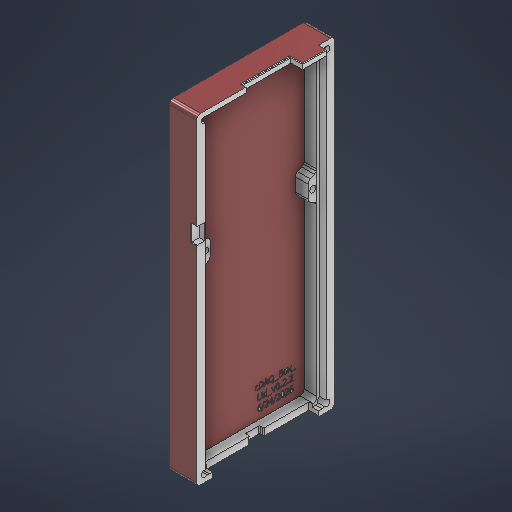
# Autodesk Inventor part: cDAQ_Box_Lid_v0.2.3
Saved by Autodesk Inventor 2027 (Build 310192000, 192)
## iProperties
Created: 2026-05-08
Part Number: cDAQ_Box_Lid_v0.2.3
Material: Generic
Document SubType Name: Modeling
Designer: giese
Density: 1 g/cm^3
Appearance: Default
Author: giese
Autodesk Inventor part; units mm, degrees
(part 1 of 2)
ref_plane "YZ Plane" through (0, 0, 0) normal (1, 0, 0) x (0, 1, 0)
ref_plane "XZ Plane" through (0, 0, 0) normal (0, 1, 0) x (-1, 0, 0)
ref_plane "XY Plane" through (0, 0, 0) normal (0, 0, 1) x (1, 0, 0)
sketch "Sketch1" plane through (0, 0, 0) normal (1, 0, 0) x (0, 1, 0)
  line L0 (50.7569, 48.4212) -> (-204.2591, 48.4212)
  line L1 (-204.2591, 48.4212) -> (-204.2591, -60.7988)
  line L2 (-204.2591, -60.7988) -> (50.7569, -60.7988)
  line L3 (50.7569, -60.7988) -> (50.7569, 48.4212)
  point P0 (0, 0)
  dimension "d0" = 109.22
  dimension "d1" = 255.016
  constraints: 8 end point, 2 parallel, 1 horizontal, 1 perpendicular
  measures "d0" distance of L2.end L0.start
  measures "d1" distance of L0.start L0.end
extrude "Extrusion1" add sketch "Sketch1" along normal blind 21.59
sketch "Sketch2" plane through (21.59, 0, 0) normal (1, 0, 0) x (0, 0, -1)
  line L0 (-39.5312, 44.4069) -> (51.9088, 44.4069)
  line L1 (51.9088, 44.4069) -> (51.9088, -197.9091)
  line L2 (51.9088, -197.9091) -> (-39.5312, -197.9091)
  line L3 (-39.5312, -197.9091) -> (-39.5312, 44.4069)
  line L4 (-48.4212, 50.7569) -> (-48.4212, -204.2591) projected
  line L5 (-48.4212, -204.2591) -> (60.7988, -204.2591) projected
  line L6 (60.7988, -204.2591) -> (60.7988, 50.7569) projected
  point P0 (0, 0)
  dimension "d4" = 91.44
  dimension "d5" = 242.316
  dimension "d6" = 8.89
  dimension "d7" = 6.35
  dimension "d226" = 8.89
  constraints: 8 end point, 2 parallel, 1 horizontal, 1 perpendicular
  measures "d4" distance of L0.start L0.end
  measures "d5" distance of L0.end L1.end
  measures "d6" distance between parallel lines of L4 L3
  measures "d7" distance between parallel lines of L5 L2
  measures "d226" distance between parallel lines of L6 L1
extrude "Extrusion2" cut sketch "Sketch2" against normal blind 15.24
sketch "Sketch3" plane through (0, 0, 0) normal (-1, 0, 0) x (0, 0, 1)
  circle A0 centre (-37.9388, 7.3229) radius 2
  line L0 (-60.7988, -204.2591) -> (-60.7988, 50.7569) projected
  line L1 (-60.7988, 50.7569) -> (48.4212, 50.7569) projected
  circle A1 centre (-19.44, 7.3229) radius 2
  circle A2 centre (-0.9411, 7.3229) radius 2
  point P0 (0, 0)
  dimension "d10" = 22.86
  dimension "d11" = 43.434
  dimension "d12" = 43.434
  dimension "d13" = 18.4988
  dimension "d14" = 4
  dimension "d15" = 4
  dimension "d16" = 43.434
  dimension "d17" = 18.4988
  dimension "d18" = 36.9976
  dimension "d21" = 4
  constraints: 3 centre point
  measures "d10" distance from line of L0 A0.centre
  measures "d11" distance from line of L1 A0.centre
  measures "d12" distance from line of L1 A1.centre
  measures "d13" distance of A0.centre A1.centre
  measures "d14" diameter of A1
  measures "d15" diameter of A2
  measures "d16" distance from line of L1 A2.centre
  measures "d17" distance of A1.centre A2.centre
  measures "d18" distance of A0.centre A2.centre
  measures "d21" diameter of A0
extrude "Extrusion3" [suppressed]
sketch "Sketch6" plane through (0, 50.7569, 48.4212) normal (0, 1, 0) x (1, 0, 0)
  line L0 (21.59, 8.89) -> (21.59, 100.33) projected
  line L1 (17.78, 39.37) -> (21.59, 39.37)
  line L2 (21.59, 39.37) -> (21.59, 96.52)
  line L3 (21.59, 96.52) -> (17.78, 96.52)
  line L4 (17.78, 96.52) -> (17.78, 39.37)
  line L5 (0, 109.22) -> (21.59, 109.22) projected
  point P0 (0, 48.4212)
  point P1 (21.59, 39.37)
  point P2 (19.685, 96.52)
  point P3 (19.685, 39.37)
  dimension "d30" = 3.81
  dimension "d32" = 12.7
  dimension "d220" = 69.85
  constraints: 8 end point, 2 midpoint, 2 parallel, 1 horizontal, 1 perpendicular, 1 point on line
  measures "d30" distance between parallel lines of L0 L4
  measures "d32" distance between parallel lines of L5 L3
  measures "d220" distance between parallel lines of L5 L1
extrude "Extrusion5" cut sketch "Sketch6" against normal blind 6.35
fillet "Fillet1" radius 3.175 4 edges at (10.795, 50.7569, -60.7988) (10.795, 50.7569, 48.4212) (10.795, -204.2591, 48.4212) (10.795, -204.2591, -60.7988)
sketch "Sketch7" plane through (21.59, 0, 0) normal (1, 0, 0) x (0, 0, -1)
  line L0 (-39.5312, -197.9091) -> (-39.5312, 44.4069) projected
  line L1 (-39.5312, 44.4069) -> (-42.3252, 44.4069)
  line L2 (-42.3252, 46.6929) -> (-41.6902, 46.6929)
  line L3 (-41.6902, 46.6929) -> (-41.6902, 51.0109)
  line L4 (-39.5312, -190.1621) -> (-39.5312, -197.9091)
  line L5 (51.9088, -197.9091) -> (-39.5312, -197.9091) projected
  line L6 (-40.4202, -200.1951) -> (-41.6902, -200.1951)
  line L7 (-41.6902, -200.1951) -> (-41.6902, -190.1621)
  line L8 (51.9088, 44.4069) -> (51.9088, -197.9091) projected
  line L9 (51.9088, -192.7021) -> (51.9088, -197.9091)
  line L10 (51.9088, -197.9091) -> (43.9078, -197.9091)
  line L11 (51.9088, -197.9091) -> (51.9088, -192.7021)
  line L12 (54.0678, -192.7021) -> (54.0678, -200.1951)
  line L13 (54.0678, -200.1951) -> (43.9078, -200.1951)
  line L14 (-39.5312, 44.4069) -> (51.9088, 44.4069) projected
  line L15 (42.0028, 44.4069) -> (51.9088, 44.4069)
  line L16 (54.0678, 48.4709) -> (54.0678, 46.6929)
  line L17 (54.0678, 46.6929) -> (42.0028, 46.6929)
  line L18 (-42.3252, 46.6929) -> (42.0028, 46.6929)
  line L19 (42.0028, 44.4069) -> (-42.3252, 44.4069)
  line L20 (54.0678, 48.4709) -> (54.0678, -192.7021)
  line L21 (44.2888, -195.2421) -> (44.2888, 44.4069)
  line L22 (43.9078, -197.9091) -> (-40.4202, -197.9091)
  line L23 (-40.4202, -200.1951) -> (43.9078, -200.1951)
  line L24 (-41.6902, -190.1621) -> (-41.6902, 51.0109)
  line L25 (-39.5312, 44.4069) -> (-39.5312, -190.1621)
  point P0 (0, 0)
  point P1 (-39.5312, 51.0109)
  point P2 (-44.2302, 48.9789)
  point P3 (51.9088, 48.4709)
  point P4 (54.0678, 46.6929)
  point P5 (-42.0712, 50.7569)
  point P6 (49.3688, 50.7569)
  point P7 (-44.2302, -190.0351)
  point P8 (51.5278, -190.0351)
  point P9 (-41.6902, 46.6929)
  dimension "d34" = 2.286
  dimension "d35" = 2.159
  dimension "d38" = 2.159
  dimension "d39" = 2.286
  dimension "d42" = 2.286
  dimension "d43" = 2.159
  dimension "d46" = 2.286
  dimension "d47" = 2.159
  constraints: 44 end point, 5 point on line, 4 parallel, 4 perpendicular, 2 collinear, 2 horizontal, 2 vertical, 6 other
  measures "d34" distance between parallel lines of L2 L1
  measures "d39" distance between parallel lines of L5 L6
  measures "d42" distance between parallel lines of L5 L13
  measures "d46" distance between parallel lines of L14 L17
extrude "Extrusion6" cut sketch "Sketch7" against normal blind 5 contours L0 L14 L8 L5 | L6 L7 L24 L18 L17 L20 L12 L13 L23
fillet "Fillet2" radius 3.175 6 edges at (11.47, 44.4069, 39.5312) (11.47, 44.4069, -51.9088) (11.47, -197.9091, 39.5312) (19.09, -200.1951, 41.6902) (11.47, -197.9091, -51.9088) (19.09, -200.1951, -54.0678)
sketch "Sketch11" plane through (16.59, 0, 0) normal (1, 0, 0) x (0, 0, -1)
  circle A0 centre (54.7028, 44.6609) radius 2.4005
  line L0 (57.6238, 50.7569) -> (48.0988, 50.7569) projected
  line L1 (60.7988, -201.0841) -> (60.7988, 47.5819) projected
  arc A1 (46.9238, 45.7719) -> (43.7488, 48.9469) centre (43.7488, 45.7719) ccw projected
  circle A2 centre (-42.3252, 44.6609) radius 2.4005
  line L2 (-48.4212, 47.5819) -> (-48.4212, -201.0841) projected
  line L3 (-9.0512, 50.7569) -> (-45.2462, 50.7569) projected
  circle A3 centre (54.7028, -198.1631) radius 2.4005
  line L4 (-45.2462, -204.2591) -> (57.6238, -204.2591) projected
  circle A4 centre (-42.3252, -198.1631) radius 2.4005
  circle A5 centre (48.7338, -50.8431) radius 2.4005
  circle A6 centre (-36.3562, -50.8431) radius 2.4005
  point P0 (0, 0)
  point P1 (45.9939, 48.017)
  point P2 (48.5528, -43.2993)
  point P3 (45.3778, -46.4743)
  point P4 (-30.4007, -42.8803)
  point P5 (-33.5757, -46.0553)
  point P6 (49.3688, 50.7569)
  point P7 (-42.0712, 50.7569)
  dimension "d58" = 4.801
  dimension "d59" = 6.096
  dimension "d60" = 6.096
  dimension "d61" = 4.801
  dimension "d62" = 4.801
  dimension "d63" = 6.096
  dimension "d64" = 6.096
  dimension "d65" = 4.801
  dimension "d66" = 6.096
  dimension "d67" = 6.096
  dimension "d76" = 6.096
  dimension "d77" = 6.096
  dimension "d114" = 4.801
  dimension "d115" = 101.6
  dimension "d116" = 12.065
  dimension "d117" = 4.801
  dimension "d118" = 101.6
  dimension "d119" = 12.065
  constraints: 6 centre point, 1 point on circle
  measures "d58" diameter of A0
  measures "d59" distance from line of L2 A2.centre
  measures "d60" distance from line of L3 A2.centre
  measures "d61" diameter of A2
  measures "d62" diameter of A3
  measures "d63" distance from line of L1 A3.centre
  measures "d64" distance from line of L4 A3.centre
  measures "d65" diameter of A4
  measures "d66" distance from line of L2 A4.centre
  measures "d67" distance from line of L4 A4.centre
  measures "d76" distance from line of L1 A0.centre
  measures "d77" distance from line of L0 A0.centre
  measures "d114" diameter of A5
  measures "d115" distance from line of A5.centre L0
  measures "d116" distance from line of L1 A5.centre
  measures "d117" diameter of A6
  measures "d118" distance from line of A6.centre L3
  measures "d119" distance from line of L2 A6.centre
extrude "Extrusion8" cut sketch "Sketch11" along normal blind 5.08 and the other way blind 17.78
sketch "Sketch13" plane through (6.35, 0, 0) normal (1, 0, 0) x (0, 0, -1)
  line L0 (15.1871, -172.5143) -> (43.1301, -172.5143) construction
  line L1 (43.1301, -172.5143) -> (43.1301, -194.7142) construction
  line L2 (43.1301, -194.7142) -> (15.1871, -194.7142) construction
  line L3 (15.1871, -194.7142) -> (15.1871, -172.5143) construction
  spline S0 degree 2 poles (14.6534, -177.2604) (14.2978, -177.2604) (13.7087, -177.0418) (13.4975, -176.8195) knots 0 0 0 1 2 2 2
  spline S1 degree 2 poles (13.4975, -176.8195) (13.2863, -176.6009) (13.0529, -175.9266) (13.0529, -175.4746) knots 0 0 0 1 2 2 2
  spline S2 degree 2 poles (13.0529, -175.4746) (13.0529, -175.0226) (13.2937, -174.3631) (13.4975, -174.1408) knots 0 0 0 1 2 2 2
  spline S3 degree 2 poles (13.4975, -174.1408) (13.7012, -173.9148) (14.3052, -173.6739) (14.6534, -173.6739) knots 0 0 0 1 2 2 2
  spline S4 degree 2 poles (14.6534, -173.6739) (14.935, -173.6739) (15.4611, -173.8333) (15.6649, -173.937) knots 0 0 0 1 2 2 2
  line L4 (15.6649, -173.937) -> (15.6649, -174.5854)
  line L5 (15.6649, -174.5854) -> (15.6316, -174.5854)
  spline S5 degree 2 poles (15.6316, -174.5854) (15.5686, -174.5335) (15.3759, -174.4001) (15.2388, -174.3297) knots 0 0 0 1 2 2 2
  spline S6 degree 2 poles (15.2388, -174.3297) (15.1166, -174.2704) (14.7905, -174.1778) (14.6423, -174.1778) knots 0 0 0 1 2 2 2
  spline S7 degree 2 poles (14.6423, -174.1778) (14.194, -174.1778) (13.6494, -174.8558) (13.6494, -175.4746) knots 0 0 0 1 2 2 2
  spline S8 degree 2 poles (13.6494, -175.4746) (13.6494, -176.0785) (14.1755, -176.7565) (14.6423, -176.7565) knots 0 0 0 1 2 2 2
  spline S9 degree 2 poles (14.6423, -176.7565) (14.9239, -176.7565) (15.4352, -176.5231) (15.6316, -176.3416) knots 0 0 0 1 2 2 2
  line L6 (15.6316, -176.3416) -> (15.6649, -176.3416)
  line L7 (15.6649, -176.3416) -> (15.6649, -176.9899)
  spline S10 degree 2 poles (15.6649, -176.9899) (15.5797, -177.0307) (15.3203, -177.1455) (15.2166, -177.1715) knots 0 0 0 1 2 2 2
  spline S11 degree 2 poles (15.2166, -177.1715) (15.0684, -177.2159) (14.835, -177.2604) (14.6534, -177.2604) knots 0 0 0 1 2 2 2
  spline S12 degree 2 poles (19.8405, -174.9003) (19.8405, -175.5264) (19.3329, -176.5342) (18.9068, -176.8158) knots 0 0 0 1 2 2 2
  spline S13 degree 2 poles (18.9068, -176.8158) (18.5585, -177.0344) (17.8435, -177.1826) (17.2877, -177.1826) knots 0 0 0 1 2 2 2
  line L8 (17.2877, -177.1826) -> (16.2355, -177.1826)
  line L9 (16.2355, -177.1826) -> (16.2355, -172.6106)
  line L10 (16.2355, -172.6106) -> (17.2766, -172.6106)
  spline S14 degree 2 poles (17.2766, -172.6106) (17.9213, -172.6106) (18.6549, -172.8033) (18.9142, -172.9737) knots 0 0 0 1 2 2 2
  spline S15 degree 2 poles (18.9142, -172.9737) (19.3551, -173.2664) (19.8405, -174.2334) (19.8405, -174.9003) knots 0 0 0 1 2 2 2
  spline S16 degree 2 poles (19.2069, -174.8929) (19.2069, -174.3668) (18.8586, -173.6221) (18.5141, -173.4109) knots 0 0 0 1 2 2 2
  spline S17 degree 2 poles (18.5141, -173.4109) (18.2695, -173.2664) (17.7175, -173.1367) (17.3062, -173.1367) knots 0 0 0 1 2 2 2
  line L11 (17.3062, -173.1367) -> (16.8431, -173.1367)
  line L12 (16.8431, -173.1367) -> (16.8431, -176.6565)
  line L13 (16.8431, -176.6565) -> (17.3062, -176.6565)
  spline S18 degree 2 poles (17.3062, -176.6565) (17.7101, -176.6565) (18.3214, -176.5268) (18.5696, -176.3527) knots 0 0 0 1 2 2 2
  spline S19 degree 2 poles (18.5696, -176.3527) (18.8883, -176.1378) (19.2069, -175.4264) (19.2069, -174.8929) knots 0 0 0 1 2 2 2
  line L14 (20.0072, -177.1826) -> (21.5485, -172.6106)
  line L15 (21.5485, -172.6106) -> (22.2969, -172.6106)
  line L16 (22.2969, -172.6106) -> (23.8382, -177.1826)
  line L17 (23.8382, -177.1826) -> (23.1972, -177.1826)
  line L18 (23.1972, -177.1826) -> (22.7823, -175.9044)
  line L19 (22.7823, -175.9044) -> (21.0372, -175.9044)
  line L20 (21.0372, -175.9044) -> (20.6222, -177.1826)
  line L21 (20.6222, -177.1826) -> (20.0072, -177.1826)
  line L22 (22.6155, -175.3857) -> (21.9079, -173.233)
  line L23 (21.9079, -173.233) -> (21.2039, -175.3857)
  line L24 (21.2039, -175.3857) -> (22.6155, -175.3857)
  spline S20 degree 2 poles (28.0693, -178.3015) (27.9026, -178.3423) (27.5395, -178.3867) (27.358, -178.3867) knots 0 0 0 1 2 2 2
  spline S21 degree 2 poles (27.358, -178.3867) (26.843, -178.3867) (26.202, -177.8124) (26.1724, -177.2789) knots 0 0 0 1 2 2 2
  spline S22 degree 2 poles (26.1724, -177.2789) (26.1316, -177.2789) (26.0612, -177.2789) (26.0316, -177.2789) knots 0 0 0 1 2 2 2
  spline S23 degree 2 poles (26.0316, -177.2789) (25.5684, -177.2789) (24.8237, -176.964) (24.557, -176.6565) knots 0 0 0 1 2 2 2
  spline S24 degree 2 poles (24.557, -176.6565) (24.2939, -176.3527) (24.0123, -175.4635) (24.0123, -174.9003) knots 0 0 0 1 2 2 2
  spline S25 degree 2 poles (24.0123, -174.9003) (24.0123, -174.3223) (24.2976, -173.4479) (24.5607, -173.1367) knots 0 0 0 1 2 2 2
  spline S26 degree 2 poles (24.5607, -173.1367) (24.8274, -172.8292) (25.5721, -172.5143) (26.0316, -172.5143) knots 0 0 0 1 2 2 2
  spline S27 degree 2 poles (26.0316, -172.5143) (26.4984, -172.5143) (27.2468, -172.8403) (27.5062, -173.1367) knots 0 0 0 1 2 2 2
  spline S28 degree 2 poles (27.5062, -173.1367) (27.7655, -173.4368) (28.0545, -174.3297) (28.0545, -174.9003) knots 0 0 0 1 2 2 2
  spline S29 degree 2 poles (28.0545, -174.9003) (28.0545, -175.7895) (27.3617, -176.9455) (26.7577, -177.1493) knots 0 0 0 1 2 2 2
  spline S30 degree 2 poles (26.7577, -177.1493) (26.7726, -177.3197) (26.8615, -177.5939) (26.9319, -177.6717) knots 0 0 0 1 2 2 2
  spline S31 degree 2 poles (26.9319, -177.6717) (27.0171, -177.768) (27.2505, -177.8569) (27.458, -177.8569) knots 0 0 0 1 2 2 2
  spline S32 degree 2 poles (27.458, -177.8569) (27.5803, -177.8569) (27.9137, -177.7791) (27.9878, -177.7495) knots 0 0 0 1 2 2 2
  line L25 (27.9878, -177.7495) -> (28.0693, -177.7495)
  line L26 (28.0693, -177.7495) -> (28.0693, -178.3015)
  spline S33 degree 2 poles (27.4209, -174.9003) (27.4209, -174.4446) (27.2246, -173.7443) (27.0467, -173.5146) knots 0 0 0 1 2 2 2
  spline S34 degree 2 poles (27.0467, -173.5146) (26.8652, -173.2775) (26.3539, -173.0404) (26.0353, -173.0404) knots 0 0 0 1 2 2 2
  spline S35 degree 2 poles (26.0353, -173.0404) (25.7055, -173.0404) (25.209, -173.2701) (25.0201, -173.5146) knots 0 0 0 1 2 2 2
  spline S36 degree 2 poles (25.0201, -173.5146) (24.8385, -173.748) (24.6459, -174.4557) (24.6459, -174.9003) knots 0 0 0 1 2 2 2
  spline S37 degree 2 poles (24.6459, -174.9003) (24.6459, -175.8006) (25.4017, -176.7602) (26.0353, -176.7602) knots 0 0 0 1 2 2 2
  spline S38 degree 2 poles (26.0353, -176.7602) (26.6688, -176.7602) (27.4209, -175.8006) (27.4209, -174.9003) knots 0 0 0 1 2 2 2
  line L27 (31.7373, -178.1014) -> (28.2101, -178.1014)
  line L28 (28.2101, -178.1014) -> (28.2101, -177.705)
  line L29 (28.2101, -177.705) -> (31.7373, -177.705)
  line L30 (31.7373, -177.705) -> (31.7373, -178.1014)
  spline S39 degree 2 poles (35.2534, -175.7784) (35.2534, -176.1193) (34.994, -176.6417) (34.7791, -176.8121) knots 0 0 0 1 2 2 2
  spline S40 degree 2 poles (34.7791, -176.8121) (34.5198, -177.0122) (33.9307, -177.1826) (33.4638, -177.1826) knots 0 0 0 1 2 2 2
  line L31 (33.4638, -177.1826) -> (32.1523, -177.1826)
  line L32 (32.1523, -177.1826) -> (32.1523, -172.6106)
  line L33 (32.1523, -172.6106) -> (33.3638, -172.6106)
  spline S41 degree 2 poles (33.3638, -172.6106) (33.8529, -172.6106) (34.3419, -172.6736) (34.5642, -172.7958) knots 0 0 0 1 2 2 2
  spline S42 degree 2 poles (34.5642, -172.7958) (34.8125, -172.9255) (35.0385, -173.3516) (35.0385, -173.6406) knots 0 0 0 1 2 2 2
  spline S43 degree 2 poles (35.0385, -173.6406) (35.0385, -173.9629) (34.6976, -174.4742) (34.3975, -174.6187) knots 0 0 0 1 2 2 2
  line L34 (34.3975, -174.6187) -> (34.3975, -174.6409)
  spline S44 degree 2 poles (34.3975, -174.6409) (34.8051, -174.7521) (35.2534, -175.3412) (35.2534, -175.7784) knots 0 0 0 1 2 2 2
  spline S45 degree 2 poles (34.6198, -175.8043) (34.6198, -175.545) (34.4716, -175.2115) (34.2493, -175.093) knots 0 0 0 1 2 2 2
  spline S46 degree 2 poles (34.2493, -175.093) (34.1048, -175.0189) (33.764, -174.9744) (33.449, -174.9744) knots 0 0 0 1 2 2 2
  line L35 (33.449, -174.9744) -> (32.7599, -174.9744)
  line L36 (32.7599, -174.9744) -> (32.7599, -176.6639)
  line L37 (32.7599, -176.6639) -> (33.2527, -176.6639)
  spline S47 degree 2 poles (33.2527, -176.6639) (33.6528, -176.6639) (34.1122, -176.5898) (34.2901, -176.4712) knots 0 0 0 1 2 2 2
  spline S48 degree 2 poles (34.2901, -176.4712) (34.4605, -176.349) (34.6198, -176.0452) (34.6198, -175.8043) knots 0 0 0 1 2 2 2
  spline S49 degree 2 poles (34.4049, -173.7258) (34.4049, -173.5628) (34.2938, -173.3183) (34.1715, -173.2479) knots 0 0 0 1 2 2 2
  spline S50 degree 2 poles (34.1715, -173.2479) (34.0233, -173.1663) (33.6639, -173.1293) (33.3416, -173.1293) knots 0 0 0 1 2 2 2
  line L38 (33.3416, -173.1293) -> (32.7599, -173.1293)
  line L39 (32.7599, -173.1293) -> (32.7599, -174.4668)
  line L40 (32.7599, -174.4668) -> (33.449, -174.4668)
  spline S51 degree 2 poles (33.449, -174.4668) (33.7343, -174.4668) (34.0048, -174.4075) (34.1493, -174.3149) knots 0 0 0 1 2 2 2
  spline S52 degree 2 poles (34.1493, -174.3149) (34.2901, -174.226) (34.4049, -173.9407) (34.4049, -173.7258) knots 0 0 0 1 2 2 2
  spline S53 degree 2 poles (38.6324, -175.4672) (38.6324, -176.3341) (37.7987, -177.2789) (37.1022, -177.2789) knots 0 0 0 1 2 2 2
  spline S54 degree 2 poles (37.1022, -177.2789) (36.3871, -177.2789) (35.5683, -176.3045) (35.5683, -175.4672) knots 0 0 0 1 2 2 2
  spline S55 degree 2 poles (35.5683, -175.4672) (35.5683, -174.6076) (36.413, -173.6554) (37.1022, -173.6554) knots 0 0 0 1 2 2 2
  spline S56 degree 2 poles (37.1022, -173.6554) (37.7987, -173.6554) (38.6324, -174.6039) (38.6324, -175.4672) knots 0 0 0 1 2 2 2
  spline S57 degree 2 poles (38.0358, -175.4672) (38.0358, -174.8003) (37.5505, -174.1519) (37.1022, -174.1519) knots 0 0 0 1 2 2 2
  spline S58 degree 2 poles (37.1022, -174.1519) (36.6539, -174.1519) (36.1648, -174.8003) (36.1648, -175.4672) knots 0 0 0 1 2 2 2
  spline S59 degree 2 poles (36.1648, -175.4672) (36.1648, -176.1155) (36.6539, -176.7825) (37.1022, -176.7825) knots 0 0 0 1 2 2 2
  spline S60 degree 2 poles (37.1022, -176.7825) (37.5468, -176.7825) (38.0358, -176.1267) (38.0358, -175.4672) knots 0 0 0 1 2 2 2
  line L41 (41.8891, -177.1826) -> (41.1814, -177.1826)
  line L42 (41.1814, -177.1826) -> (40.3478, -175.8932)
  line L43 (40.3478, -175.8932) -> (39.4919, -177.1826)
  line L44 (39.4919, -177.1826) -> (38.8361, -177.1826)
  line L45 (38.8361, -177.1826) -> (40.0254, -175.482)
  line L46 (40.0254, -175.482) -> (38.8472, -173.7517)
  line L47 (38.8472, -173.7517) -> (39.5549, -173.7517)
  line L48 (39.5549, -173.7517) -> (40.3848, -175.03)
  line L49 (40.3848, -175.03) -> (41.2333, -173.7517)
  line L50 (41.2333, -173.7517) -> (41.8891, -173.7517)
  line L51 (41.8891, -173.7517) -> (40.7072, -175.4449)
  line L52 (40.7072, -175.4449) -> (41.8891, -177.1826)
  line L53 (45.3977, -178.1014) -> (41.8705, -178.1014)
  line L54 (41.8705, -178.1014) -> (41.8705, -177.705)
  line L55 (41.8705, -177.705) -> (45.3977, -177.705)
  line L56 (45.3977, -177.705) -> (45.3977, -178.1014)
  line L57 (17.9194, -184.7103) -> (15.2703, -184.7103)
  line L58 (15.2703, -184.7103) -> (15.2703, -180.1383)
  line L59 (15.2703, -180.1383) -> (15.8779, -180.1383)
  line L60 (15.8779, -180.1383) -> (15.8779, -184.1693)
  line L61 (15.8779, -184.1693) -> (17.9194, -184.1693)
  line L62 (17.9194, -184.1693) -> (17.9194, -184.7103)
  line L63 (18.942, -184.7103) -> (18.364, -184.7103)
  line L64 (18.364, -184.7103) -> (18.364, -181.2794)
  line L65 (18.364, -181.2794) -> (18.942, -181.2794)
  line L66 (18.942, -181.2794) -> (18.942, -184.7103)
  line L67 (18.9828, -180.7088) -> (18.327, -180.7088)
  line L68 (18.327, -180.7088) -> (18.327, -180.1086)
  line L69 (18.327, -180.1086) -> (18.9828, -180.1086)
  line L70 (18.9828, -180.1086) -> (18.9828, -180.7088)
  line L71 (22.4284, -184.7103) -> (21.8504, -184.7103)
  line L72 (21.8504, -184.7103) -> (21.8504, -184.362)
  spline S61 degree 2 poles (21.8504, -184.362) (21.7171, -184.4732) (21.5207, -184.6214) (21.3873, -184.6843) knots 0 0 0 1 2 2 2
  spline S62 degree 2 poles (21.3873, -184.6843) (21.2651, -184.7436) (21.002, -184.8066) (20.8279, -184.8066) knots 0 0 0 1 2 2 2
  spline S63 degree 2 poles (20.8279, -184.8066) (20.5463, -184.8066) (20.072, -184.5732) (19.9053, -184.3472) knots 0 0 0 1 2 2 2
  spline S64 degree 2 poles (19.9053, -184.3472) (19.7386, -184.1212) (19.5533, -183.4543) (19.5533, -183.0208) knots 0 0 0 1 2 2 2
  spline S65 degree 2 poles (19.5533, -183.0208) (19.5533, -182.5688) (19.7867, -181.9093) (19.9905, -181.661) knots 0 0 0 1 2 2 2
  spline S66 degree 2 poles (19.9905, -181.661) (20.1795, -181.4387) (20.7093, -181.1831) (21.002, -181.1831) knots 0 0 0 1 2 2 2
  spline S67 degree 2 poles (21.002, -181.1831) (21.2576, -181.1831) (21.6393, -181.2979) (21.8504, -181.4165) knots 0 0 0 1 2 2 2
  line L73 (21.8504, -181.4165) -> (21.8504, -179.9345)
  line L74 (21.8504, -179.9345) -> (22.4284, -179.9345)
  line L75 (22.4284, -179.9345) -> (22.4284, -184.7103)
  line L76 (21.8504, -183.8766) -> (21.8504, -181.8945)
  spline S68 degree 2 poles (21.8504, -181.8945) (21.6356, -181.7907) (21.2947, -181.7129) (21.0983, -181.7129) knots 0 0 0 1 2 2 2
  spline S69 degree 2 poles (21.0983, -181.7129) (20.6537, -181.7129) (20.1498, -182.3798) (20.1498, -183.0097) knots 0 0 0 1 2 2 2
  spline S70 degree 2 poles (20.1498, -183.0097) (20.1498, -183.6173) (20.5352, -184.2583) (20.9612, -184.2583) knots 0 0 0 1 2 2 2
  spline S71 degree 2 poles (20.9612, -184.2583) (21.1872, -184.2583) (21.6467, -184.0508) (21.8504, -183.8766) knots 0 0 0 1 2 2 2
  line L77 (26.3261, -185.6291) -> (22.7989, -185.6291)
  line L78 (22.7989, -185.6291) -> (22.7989, -185.2327)
  line L79 (22.7989, -185.2327) -> (26.3261, -185.2327)
  line L80 (26.3261, -185.2327) -> (26.3261, -185.6291)
  line L81 (29.3902, -181.2794) -> (28.0971, -184.7103)
  line L82 (28.0971, -184.7103) -> (27.5784, -184.7103)
  line L83 (27.5784, -184.7103) -> (26.2965, -181.2794)
  line L84 (26.2965, -181.2794) -> (26.9226, -181.2794)
  line L85 (26.9226, -181.2794) -> (27.86, -183.9211)
  line L86 (27.86, -183.9211) -> (28.79, -181.2794)
  line L87 (28.79, -181.2794) -> (29.3902, -181.2794)
  spline S72 degree 2 poles (32.5876, -182.4243) (32.5876, -183.6543) (31.8725, -184.8066) (31.1278, -184.8066) knots 0 0 0 1 2 2 2
  spline S73 degree 2 poles (31.1278, -184.8066) (30.372, -184.8066) (29.6643, -183.6321) (29.6643, -182.428) knots 0 0 0 1 2 2 2
  spline S74 degree 2 poles (29.6643, -182.428) (29.6643, -181.1905) (30.3794, -180.0456) (31.1278, -180.0456) knots 0 0 0 1 2 2 2
  spline S75 degree 2 poles (31.1278, -180.0456) (31.8799, -180.0456) (32.5876, -181.2313) (32.5876, -182.4243) knots 0 0 0 1 2 2 2
  spline S76 degree 2 poles (31.8021, -183.8174) (31.8911, -183.5914) (31.9652, -182.8948) (31.9652, -182.4243) knots 0 0 0 1 2 2 2
  spline S77 degree 2 poles (31.9652, -182.4243) (31.9652, -181.9537) (31.8911, -181.2609) (31.7984, -181.0275) knots 0 0 0 1 2 2 2
  spline S78 degree 2 poles (31.7984, -181.0275) (31.7058, -180.7941) (31.3835, -180.5532) (31.1278, -180.5532) knots 0 0 0 1 2 2 2
  spline S79 degree 2 poles (31.1278, -180.5532) (30.8722, -180.5532) (30.5424, -180.7941) (30.4461, -181.0349) knots 0 0 0 1 2 2 2
  spline S80 degree 2 poles (30.4461, -181.0349) (30.3535, -181.2683) (30.2868, -181.9797) (30.2868, -182.428) knots 0 0 0 1 2 2 2
  spline S81 degree 2 poles (30.2868, -182.428) (30.2868, -182.9096) (30.3461, -183.5543) (30.4424, -183.8062) knots 0 0 0 1 2 2 2
  spline S82 degree 2 poles (30.4424, -183.8062) (30.5313, -184.0434) (30.8611, -184.299) (31.1278, -184.299) knots 0 0 0 1 2 2 2
  spline S83 degree 2 poles (31.1278, -184.299) (31.3798, -184.299) (31.7095, -184.0582) (31.8021, -183.8174) knots 0 0 0 1 2 2 2
  line L88 (34.1548, -184.7103) -> (33.4212, -184.7103)
  line L89 (33.4212, -184.7103) -> (33.4212, -183.8359)
  line L90 (33.4212, -183.8359) -> (34.1548, -183.8359)
  line L91 (34.1548, -183.8359) -> (34.1548, -184.7103)
  line L92 (37.8969, -184.7103) -> (35.0774, -184.7103)
  line L93 (35.0774, -184.7103) -> (35.0774, -184.0619)
  spline S84 degree 2 poles (35.0774, -184.0619) (35.3812, -183.7766) (35.9221, -183.2468) (36.1815, -182.9615) knots 0 0 0 1 2 2 2
  spline S85 degree 2 poles (36.1815, -182.9615) (36.7039, -182.3872) (37.0855, -181.6981) (37.0855, -181.3313) knots 0 0 0 1 2 2 2
  spline S86 degree 2 poles (37.0855, -181.3313) (37.0855, -181.1386) (36.9669, -180.8496) (36.8595, -180.757) knots 0 0 0 1 2 2 2
  spline S87 degree 2 poles (36.8595, -180.757) (36.7521, -180.6644) (36.4705, -180.5718) (36.3, -180.5718) knots 0 0 0 1 2 2 2
  spline S88 degree 2 poles (36.3, -180.5718) (36.137, -180.5718) (35.8036, -180.6533) (35.6517, -180.7163) knots 0 0 0 1 2 2 2
  spline S89 degree 2 poles (35.6517, -180.7163) (35.522, -180.7681) (35.2812, -180.9163) (35.2071, -180.9682) knots 0 0 0 1 2 2 2
  line L94 (35.2071, -180.9682) -> (35.1737, -180.9682)
  line L95 (35.1737, -180.9682) -> (35.1737, -180.3161)
  spline S90 degree 2 poles (35.1737, -180.3161) (35.3627, -180.2235) (36.0407, -180.0419) (36.3445, -180.0419) knots 0 0 0 1 2 2 2
  spline S91 degree 2 poles (36.3445, -180.0419) (36.9855, -180.0419) (37.7079, -180.72) (37.7079, -181.2979) knots 0 0 0 1 2 2 2
  spline S92 degree 2 poles (37.7079, -181.2979) (37.7079, -181.5684) (37.582, -182.0204) (37.4708, -182.2131) knots 0 0 0 1 2 2 2
  spline S93 degree 2 poles (37.4708, -182.2131) (37.3597, -182.4132) (37.0373, -182.8059) (36.8595, -182.9948) knots 0 0 0 1 2 2 2
  spline S94 degree 2 poles (36.8595, -182.9948) (36.5705, -183.3098) (35.8628, -183.9841) (35.6517, -184.1805) knots 0 0 0 1 2 2 2
  line L96 (35.6517, -184.1805) -> (37.8969, -184.1805)
  line L97 (37.8969, -184.1805) -> (37.8969, -184.7103)
  line L98 (39.4901, -184.7103) -> (38.7565, -184.7103)
  line L99 (38.7565, -184.7103) -> (38.7565, -183.8359)
  line L100 (38.7565, -183.8359) -> (39.4901, -183.8359)
  line L101 (39.4901, -183.8359) -> (39.4901, -184.7103)
  line L102 (43.2321, -184.7103) -> (40.4126, -184.7103)
  line L103 (40.4126, -184.7103) -> (40.4126, -184.0619)
  spline S95 degree 2 poles (40.4126, -184.0619) (40.7164, -183.7766) (41.2574, -183.2468) (41.5167, -182.9615) knots 0 0 0 1 2 2 2
  spline S96 degree 2 poles (41.5167, -182.9615) (42.0391, -182.3872) (42.4207, -181.6981) (42.4207, -181.3313) knots 0 0 0 1 2 2 2
  spline S97 degree 2 poles (42.4207, -181.3313) (42.4207, -181.1386) (42.3022, -180.8496) (42.1947, -180.757) knots 0 0 0 1 2 2 2
  spline S98 degree 2 poles (42.1947, -180.757) (42.0873, -180.6644) (41.8057, -180.5718) (41.6353, -180.5718) knots 0 0 0 1 2 2 2
  spline S99 degree 2 poles (41.6353, -180.5718) (41.4723, -180.5718) (41.1388, -180.6533) (40.9869, -180.7163) knots 0 0 0 1 2 2 2
  spline S100 degree 2 poles (40.9869, -180.7163) (40.8572, -180.7681) (40.6164, -180.9163) (40.5423, -180.9682) knots 0 0 0 1 2 2 2
  line L104 (40.5423, -180.9682) -> (40.5089, -180.9682)
  line L105 (40.5089, -180.9682) -> (40.5089, -180.3161)
  spline S101 degree 2 poles (40.5089, -180.3161) (40.6979, -180.2235) (41.3759, -180.0419) (41.6797, -180.0419) knots 0 0 0 1 2 2 2
  spline S102 degree 2 poles (41.6797, -180.0419) (42.3207, -180.0419) (43.0432, -180.72) (43.0432, -181.2979) knots 0 0 0 1 2 2 2
  spline S103 degree 2 poles (43.0432, -181.2979) (43.0432, -181.5684) (42.9172, -182.0204) (42.8061, -182.2131) knots 0 0 0 1 2 2 2
  spline S104 degree 2 poles (42.8061, -182.2131) (42.6949, -182.4132) (42.3726, -182.8059) (42.1947, -182.9948) knots 0 0 0 1 2 2 2
  spline S105 degree 2 poles (42.1947, -182.9948) (41.9057, -183.3098) (41.1981, -183.9841) (40.9869, -184.1805) knots 0 0 0 1 2 2 2
  line L106 (40.9869, -184.1805) -> (43.2321, -184.1805)
  line L107 (43.2321, -184.1805) -> (43.2321, -184.7103)
  spline S106 degree 2 poles (17.9694, -190.7559) (17.9694, -191.1079) (17.736, -191.7044) (17.5396, -191.9045) knots 0 0 0 1 2 2 2
  spline S107 degree 2 poles (17.5396, -191.9045) (17.3359, -192.1157) (16.8246, -192.3343) (16.5171, -192.3343) knots 0 0 0 1 2 2 2
  spline S108 degree 2 poles (16.5171, -192.3343) (16.2095, -192.3343) (15.702, -192.1268) (15.5093, -191.9193) knots 0 0 0 1 2 2 2
  spline S109 degree 2 poles (15.5093, -191.9193) (15.2722, -191.6711) (15.0054, -190.8375) (15.0054, -190.2298) knots 0 0 0 1 2 2 2
  spline S110 degree 2 poles (15.0054, -190.2298) (15.0054, -189.6333) (15.2499, -188.6737) (15.5056, -188.318) knots 0 0 0 1 2 2 2
  spline S111 degree 2 poles (15.5056, -188.318) (15.7538, -187.9698) (16.5393, -187.5807) (17.0543, -187.5807) knots 0 0 0 1 2 2 2
  spline S112 degree 2 poles (17.0543, -187.5807) (17.2062, -187.5807) (17.473, -187.6104) (17.573, -187.6437) knots 0 0 0 1 2 2 2
  line L108 (17.573, -187.6437) -> (17.573, -188.2328)
  line L109 (17.573, -188.2328) -> (17.5471, -188.2328)
  spline S113 degree 2 poles (17.5471, -188.2328) (17.4618, -188.1884) (17.1506, -188.1106) (16.9728, -188.1106) knots 0 0 0 1 2 2 2
  spline S114 degree 2 poles (16.9728, -188.1106) (16.4022, -188.1106) (15.702, -188.8812) (15.6353, -189.637) knots 0 0 0 1 2 2 2
  spline S115 degree 2 poles (15.6353, -189.637) (15.8539, -189.4851) (16.3133, -189.3184) (16.5875, -189.3184) knots 0 0 0 1 2 2 2
  spline S116 degree 2 poles (16.5875, -189.3184) (16.8542, -189.3184) (17.2544, -189.4258) (17.473, -189.5889) knots 0 0 0 1 2 2 2
  spline S117 degree 2 poles (17.473, -189.5889) (17.7249, -189.7778) (17.9694, -190.3632) (17.9694, -190.7559) knots 0 0 0 1 2 2 2
  spline S118 degree 2 poles (17.347, -190.7819) (17.347, -190.5003) (17.1988, -190.1187) (17.0358, -189.9853) knots 0 0 0 1 2 2 2
  spline S119 degree 2 poles (17.0358, -189.9853) (16.9135, -189.889) (16.6097, -189.826) (16.4504, -189.826) knots 0 0 0 1 2 2 2
  spline S120 degree 2 poles (16.4504, -189.826) (16.2355, -189.826) (15.8316, -189.9557) (15.6353, -190.0779) knots 0 0 0 1 2 2 2
  spline S121 degree 2 poles (15.6353, -190.0779) (15.6316, -190.1446) (15.6242, -190.2706) (15.6242, -190.3669) knots 0 0 0 1 2 2 2
  spline S122 degree 2 poles (15.6242, -190.3669) (15.6242, -190.8412) (15.8094, -191.4228) (15.9502, -191.5748) knots 0 0 0 1 2 2 2
  spline S123 degree 2 poles (15.9502, -191.5748) (16.0799, -191.7192) (16.3615, -191.8341) (16.5208, -191.8341) knots 0 0 0 1 2 2 2
  spline S124 degree 2 poles (16.5208, -191.8341) (16.8913, -191.8341) (17.347, -191.308) (17.347, -190.7819) knots 0 0 0 1 2 2 2
  line L110 (20.411, -187.4622) -> (18.6215, -193.2309)
  line L111 (18.6215, -193.2309) -> (18.1028, -193.2309)
  line L112 (18.1028, -193.2309) -> (19.8849, -187.4622)
  line L113 (19.8849, -187.4622) -> (20.411, -187.4622)
  line L114 (23.7345, -192.238) -> (20.9149, -192.238)
  line L115 (20.9149, -192.238) -> (20.9149, -191.5896)
  spline S125 degree 2 poles (20.9149, -191.5896) (21.2187, -191.3043) (21.7597, -190.7745) (22.019, -190.4892) knots 0 0 0 1 2 2 2
  spline S126 degree 2 poles (22.019, -190.4892) (22.5414, -189.9149) (22.9231, -189.2258) (22.9231, -188.859) knots 0 0 0 1 2 2 2
  spline S127 degree 2 poles (22.9231, -188.859) (22.9231, -188.6663) (22.8045, -188.3773) (22.697, -188.2847) knots 0 0 0 1 2 2 2
  spline S128 degree 2 poles (22.697, -188.2847) (22.5896, -188.1921) (22.308, -188.0994) (22.1376, -188.0994) knots 0 0 0 1 2 2 2
  spline S129 degree 2 poles (22.1376, -188.0994) (21.9746, -188.0994) (21.6411, -188.1809) (21.4892, -188.2439) knots 0 0 0 1 2 2 2
  spline S130 degree 2 poles (21.4892, -188.2439) (21.3595, -188.2958) (21.1187, -188.444) (21.0446, -188.4959) knots 0 0 0 1 2 2 2
  line L116 (21.0446, -188.4959) -> (21.0113, -188.4959)
  line L117 (21.0113, -188.4959) -> (21.0113, -187.8438)
  spline S131 degree 2 poles (21.0113, -187.8438) (21.2002, -187.7512) (21.8782, -187.5696) (22.182, -187.5696) knots 0 0 0 1 2 2 2
  spline S132 degree 2 poles (22.182, -187.5696) (22.823, -187.5696) (23.5455, -188.2476) (23.5455, -188.8256) knots 0 0 0 1 2 2 2
  spline S133 degree 2 poles (23.5455, -188.8256) (23.5455, -189.0961) (23.4195, -189.5481) (23.3084, -189.7408) knots 0 0 0 1 2 2 2
  spline S134 degree 2 poles (23.3084, -189.7408) (23.1972, -189.9408) (22.8749, -190.3336) (22.697, -190.5225) knots 0 0 0 1 2 2 2
  spline S135 degree 2 poles (22.697, -190.5225) (22.4081, -190.8375) (21.7004, -191.5118) (21.4892, -191.7081) knots 0 0 0 1 2 2 2
  line L118 (21.4892, -191.7081) -> (23.7345, -191.7081)
  line L119 (23.7345, -191.7081) -> (23.7345, -192.238)
  line L120 (27.2876, -190.667) -> (26.7429, -190.667)
  line L121 (26.7429, -190.667) -> (26.7429, -192.238)
  line L122 (26.7429, -192.238) -> (26.1538, -192.238)
  line L123 (26.1538, -192.238) -> (26.1538, -190.667)
  line L124 (26.1538, -190.667) -> (24.1346, -190.667)
  line L125 (24.1346, -190.667) -> (24.1346, -190.0223)
  line L126 (24.1346, -190.0223) -> (26.1798, -187.666)
  line L127 (26.1798, -187.666) -> (26.7429, -187.666)
  line L128 (26.7429, -187.666) -> (26.7429, -190.1743)
  line L129 (26.7429, -190.1743) -> (27.2876, -190.1743)
  line L130 (27.2876, -190.1743) -> (27.2876, -190.667)
  line L131 (26.1538, -190.1743) -> (26.1538, -188.3884)
  line L132 (26.1538, -188.3884) -> (24.6162, -190.1743)
  line L133 (24.6162, -190.1743) -> (26.1538, -190.1743)
  line L134 (29.6773, -187.4622) -> (27.8878, -193.2309)
  line L135 (27.8878, -193.2309) -> (27.3691, -193.2309)
  line L136 (27.3691, -193.2309) -> (29.1512, -187.4622)
  line L137 (29.1512, -187.4622) -> (29.6773, -187.4622)
  line L138 (33.0007, -192.238) -> (30.1812, -192.238)
  line L139 (30.1812, -192.238) -> (30.1812, -191.5896)
  spline S136 degree 2 poles (30.1812, -191.5896) (30.485, -191.3043) (31.0259, -190.7745) (31.2853, -190.4892) knots 0 0 0 1 2 2 2
  spline S137 degree 2 poles (31.2853, -190.4892) (31.8077, -189.9149) (32.1893, -189.2258) (32.1893, -188.859) knots 0 0 0 1 2 2 2
  spline S138 degree 2 poles (32.1893, -188.859) (32.1893, -188.6663) (32.0708, -188.3773) (31.9633, -188.2847) knots 0 0 0 1 2 2 2
  spline S139 degree 2 poles (31.9633, -188.2847) (31.8559, -188.1921) (31.5743, -188.0994) (31.4039, -188.0994) knots 0 0 0 1 2 2 2
  spline S140 degree 2 poles (31.4039, -188.0994) (31.2408, -188.0994) (30.9074, -188.1809) (30.7555, -188.2439) knots 0 0 0 1 2 2 2
  spline S141 degree 2 poles (30.7555, -188.2439) (30.6258, -188.2958) (30.385, -188.444) (30.3109, -188.4959) knots 0 0 0 1 2 2 2
  line L140 (30.3109, -188.4959) -> (30.2775, -188.4959)
  line L141 (30.2775, -188.4959) -> (30.2775, -187.8438)
  spline S142 degree 2 poles (30.2775, -187.8438) (30.4665, -187.7512) (31.1445, -187.5696) (31.4483, -187.5696) knots 0 0 0 1 2 2 2
  spline S143 degree 2 poles (31.4483, -187.5696) (32.0893, -187.5696) (32.8118, -188.2476) (32.8118, -188.8256) knots 0 0 0 1 2 2 2
  spline S144 degree 2 poles (32.8118, -188.8256) (32.8118, -189.0961) (32.6858, -189.5481) (32.5746, -189.7408) knots 0 0 0 1 2 2 2
  spline S145 degree 2 poles (32.5746, -189.7408) (32.4635, -189.9408) (32.1412, -190.3336) (31.9633, -190.5225) knots 0 0 0 1 2 2 2
  spline S146 degree 2 poles (31.9633, -190.5225) (31.6743, -190.8375) (30.9667, -191.5118) (30.7555, -191.7081) knots 0 0 0 1 2 2 2
  line L142 (30.7555, -191.7081) -> (33.0007, -191.7081)
  line L143 (33.0007, -191.7081) -> (33.0007, -192.238)
  spline S147 degree 2 poles (36.4575, -189.952) (36.4575, -191.182) (35.7424, -192.3343) (34.9977, -192.3343) knots 0 0 0 1 2 2 2
  spline S148 degree 2 poles (34.9977, -192.3343) (34.2419, -192.3343) (33.5342, -191.1598) (33.5342, -189.9557) knots 0 0 0 1 2 2 2
  spline S149 degree 2 poles (33.5342, -189.9557) (33.5342, -188.7182) (34.2493, -187.5733) (34.9977, -187.5733) knots 0 0 0 1 2 2 2
  spline S150 degree 2 poles (34.9977, -187.5733) (35.7498, -187.5733) (36.4575, -188.7589) (36.4575, -189.952) knots 0 0 0 1 2 2 2
  spline S151 degree 2 poles (35.672, -191.345) (35.761, -191.119) (35.8351, -190.4225) (35.8351, -189.952) knots 0 0 0 1 2 2 2
  spline S152 degree 2 poles (35.8351, -189.952) (35.8351, -189.4814) (35.761, -188.7886) (35.6683, -188.5552) knots 0 0 0 1 2 2 2
  spline S153 degree 2 poles (35.6683, -188.5552) (35.5757, -188.3217) (35.2534, -188.0809) (34.9977, -188.0809) knots 0 0 0 1 2 2 2
  spline S154 degree 2 poles (34.9977, -188.0809) (34.7421, -188.0809) (34.4123, -188.3217) (34.316, -188.5626) knots 0 0 0 1 2 2 2
  spline S155 degree 2 poles (34.316, -188.5626) (34.2234, -188.796) (34.1567, -189.5073) (34.1567, -189.9557) knots 0 0 0 1 2 2 2
  spline S156 degree 2 poles (34.1567, -189.9557) (34.1567, -190.4373) (34.216, -191.082) (34.3123, -191.3339) knots 0 0 0 1 2 2 2
  spline S157 degree 2 poles (34.3123, -191.3339) (34.4012, -191.571) (34.731, -191.8267) (34.9977, -191.8267) knots 0 0 0 1 2 2 2
  spline S158 degree 2 poles (34.9977, -191.8267) (35.2497, -191.8267) (35.5794, -191.5859) (35.672, -191.345) knots 0 0 0 1 2 2 2
  line L144 (39.8624, -192.238) -> (37.0429, -192.238)
  line L145 (37.0429, -192.238) -> (37.0429, -191.5896)
  spline S159 degree 2 poles (37.0429, -191.5896) (37.3467, -191.3043) (37.8876, -190.7745) (38.147, -190.4892) knots 0 0 0 1 2 2 2
  spline S160 degree 2 poles (38.147, -190.4892) (38.6694, -189.9149) (39.051, -189.2258) (39.051, -188.859) knots 0 0 0 1 2 2 2
  spline S161 degree 2 poles (39.051, -188.859) (39.051, -188.6663) (38.9325, -188.3773) (38.825, -188.2847) knots 0 0 0 1 2 2 2
  spline S162 degree 2 poles (38.825, -188.2847) (38.7176, -188.1921) (38.436, -188.0994) (38.2656, -188.0994) knots 0 0 0 1 2 2 2
  spline S163 degree 2 poles (38.2656, -188.0994) (38.1025, -188.0994) (37.7691, -188.1809) (37.6172, -188.2439) knots 0 0 0 1 2 2 2
  spline S164 degree 2 poles (37.6172, -188.2439) (37.4875, -188.2958) (37.2467, -188.444) (37.1726, -188.4959) knots 0 0 0 1 2 2 2
  line L146 (37.1726, -188.4959) -> (37.1392, -188.4959)
  line L147 (37.1392, -188.4959) -> (37.1392, -187.8438)
  spline S165 degree 2 poles (37.1392, -187.8438) (37.3282, -187.7512) (38.0062, -187.5696) (38.31, -187.5696) knots 0 0 0 1 2 2 2
  spline S166 degree 2 poles (38.31, -187.5696) (38.951, -187.5696) (39.6735, -188.2476) (39.6735, -188.8256) knots 0 0 0 1 2 2 2
  spline S167 degree 2 poles (39.6735, -188.8256) (39.6735, -189.0961) (39.5475, -189.5481) (39.4363, -189.7408) knots 0 0 0 1 2 2 2
  spline S168 degree 2 poles (39.4363, -189.7408) (39.3252, -189.9408) (39.0029, -190.3336) (38.825, -190.5225) knots 0 0 0 1 2 2 2
  spline S169 degree 2 poles (38.825, -190.5225) (38.536, -190.8375) (37.8284, -191.5118) (37.6172, -191.7081) knots 0 0 0 1 2 2 2
  line L148 (37.6172, -191.7081) -> (39.8624, -191.7081)
  line L149 (39.8624, -191.7081) -> (39.8624, -192.238)
  spline S170 degree 2 poles (43.3637, -190.7559) (43.3637, -191.1079) (43.1303, -191.7044) (42.9339, -191.9045) knots 0 0 0 1 2 2 2
  spline S171 degree 2 poles (42.9339, -191.9045) (42.7301, -192.1157) (42.2188, -192.3343) (41.9113, -192.3343) knots 0 0 0 1 2 2 2
  spline S172 degree 2 poles (41.9113, -192.3343) (41.6038, -192.3343) (41.0962, -192.1268) (40.9035, -191.9193) knots 0 0 0 1 2 2 2
  spline S173 degree 2 poles (40.9035, -191.9193) (40.6664, -191.6711) (40.3996, -190.8375) (40.3996, -190.2298) knots 0 0 0 1 2 2 2
  spline S174 degree 2 poles (40.3996, -190.2298) (40.3996, -189.6333) (40.6442, -188.6737) (40.8998, -188.318) knots 0 0 0 1 2 2 2
  spline S175 degree 2 poles (40.8998, -188.318) (41.1481, -187.9698) (41.9335, -187.5807) (42.4485, -187.5807) knots 0 0 0 1 2 2 2
  spline S176 degree 2 poles (42.4485, -187.5807) (42.6004, -187.5807) (42.8672, -187.6104) (42.9672, -187.6437) knots 0 0 0 1 2 2 2
  line L150 (42.9672, -187.6437) -> (42.9672, -188.2328)
  line L151 (42.9672, -188.2328) -> (42.9413, -188.2328)
  spline S177 degree 2 poles (42.9413, -188.2328) (42.8561, -188.1884) (42.5449, -188.1106) (42.367, -188.1106) knots 0 0 0 1 2 2 2
  spline S178 degree 2 poles (42.367, -188.1106) (41.7964, -188.1106) (41.0962, -188.8812) (41.0295, -189.637) knots 0 0 0 1 2 2 2
  spline S179 degree 2 poles (41.0295, -189.637) (41.2481, -189.4851) (41.7075, -189.3184) (41.9817, -189.3184) knots 0 0 0 1 2 2 2
  spline S180 degree 2 poles (41.9817, -189.3184) (42.2485, -189.3184) (42.6486, -189.4258) (42.8672, -189.5889) knots 0 0 0 1 2 2 2
  spline S181 degree 2 poles (42.8672, -189.5889) (43.1191, -189.7778) (43.3637, -190.3632) (43.3637, -190.7559) knots 0 0 0 1 2 2 2
  spline S182 degree 2 poles (42.7412, -190.7819) (42.7412, -190.5003) (42.593, -190.1187) (42.43, -189.9853) knots 0 0 0 1 2 2 2
  spline S183 degree 2 poles (42.43, -189.9853) (42.3077, -189.889) (42.0039, -189.826) (41.8446, -189.826) knots 0 0 0 1 2 2 2
  spline S184 degree 2 poles (41.8446, -189.826) (41.6297, -189.826) (41.2259, -189.9557) (41.0295, -190.0779) knots 0 0 0 1 2 2 2
  spline S185 degree 2 poles (41.0295, -190.0779) (41.0258, -190.1446) (41.0184, -190.2706) (41.0184, -190.3669) knots 0 0 0 1 2 2 2
  spline S186 degree 2 poles (41.0184, -190.3669) (41.0184, -190.8412) (41.2036, -191.4228) (41.3444, -191.5748) knots 0 0 0 1 2 2 2
  spline S187 degree 2 poles (41.3444, -191.5748) (41.4741, -191.7192) (41.7557, -191.8341) (41.915, -191.8341) knots 0 0 0 1 2 2 2
  spline S188 degree 2 poles (41.915, -191.8341) (42.2855, -191.8341) (42.7412, -191.308) (42.7412, -190.7819) knots 0 0 0 1 2 2 2
  point P0 (0, 0)
  constraints: 2 other
emboss "Emboss1" sketch "Sketch13" operation cut depth 2.54 direction (-1, 0, 0)